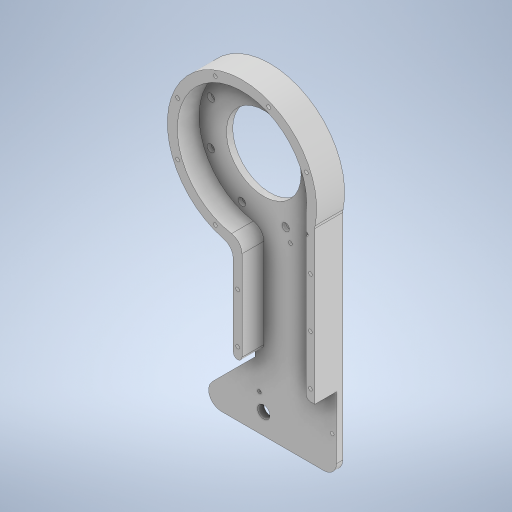
# Autodesk Inventor part: l_r_w2k_l__legparts_08(six)
Saved by Autodesk Inventor 2024.3 (Build 283343000, 343)
## iProperties
Created: 2024-10-20
Part Number: l_r_w2k_l__legparts_08(six)
Material: 一般
Document SubType Name: Modeling
Designer: 佐藤智貴
Density: 1 g/cm^3
Appearance: 既定
Mass: 466.511 g
Surface Area: 676.478 cm^2
Volume: 172.782 cm^3
Author: 佐藤智貴
Autodesk Inventor part; units mm, degrees
ref_plane "YZ Plane" through (0, 0, 0) normal (1, 0, 0) x (0, 1, 0)
ref_plane "XZ Plane" through (0, 0, 0) normal (0, 1, 0) x (-1, 0, 0)
ref_plane "XY Plane" through (0, 0, 0) normal (0, 0, 1) x (1, 0, 0)
sketch "スケッチ1" plane through (0, 0, 0) normal (0, 0, 1) x (1, 0, 0)
  circle A0 centre (0, 0) radius 60
  circle A1 centre (0, 0) radius 7
  dimension "d0" = 120
  dimension "d1" = 14
  constraints: 2 centre point, 1 coincident
  measures "d0" diameter of A0
  measures "d1" diameter of A1
extrude "押し出し1" add sketch "スケッチ1" along normal blind 5
sketch "スケッチ2" plane through (0, 0, 5) normal (0, 0, 1) x (1, 0, 0)
  circle A0 centre (0, 0) radius 46
  line L0 (0, 0) -> (0, 59.211)
  line L1 (0, 0) -> (-21.8609, 52.777)
  line L2 (0, 0) -> (27.8226, 47.8581)
  point P0 (-17.6034, 42.4985)
  point P1 (-42.4985, 17.6034)
  point P2 (-42.4985, -17.6034)
  point P3 (-17.6034, -42.4985)
  point P4 (17.6034, -42.4985)
  point P5 (42.4985, -17.6034)
  point P6 (42.4985, 17.6034)
  point P7 (17.6034, 42.4985)
  dimension "d4" = 92
  dimension "d5" = 22.5
  dimension "d8" = 360
  constraints: 6 end point, 1 coincident, 1 point on line, 1 vertical, 12 other
  measures "d5" angle of L1 L0
hole "穴1" at (-17.6034, 42.4985, 5) at (-42.4985, 17.6034, 5) at (-42.4985, -17.6034, 5) at (-17.6034, -42.4985, 5) at (17.6034, -42.4985, 5) at (42.4985, -17.6034, 5) at (42.4985, 17.6034, 5) at (17.6034, 42.4985, 5) direction (0, 0, -1) diameter 2.459 end through all
sketch "スケッチ4" plane through (0, 0, 0) normal (0, 0, -1) x (-1, 0, 0)
  line L0 (0, 0) -> (0, -80.557)
  circle A0 centre (0, 0) radius 60 projected
  line L1 (-58.5, 13.3323) -> (-58.5, -196.6677)
  line L2 (58.5, 13.3323) -> (58.5, -196.6677)
  line L3 (-58.5, -196.6677) -> (58.5, -196.6677)
  line L4 (-58.5, 13.3323) -> (-40.1274, -196.6677)
  line L5 (58.5, 13.3323) -> (40.1274, -196.6677)
  line L6 (11.2278, -149.3955) -> (58.5, -196.6677)
  line L7 (18.206, -156.3737) -> (-9.1224, -129.0453)
  line L8 (0, -80.557) -> (0, -138.1677)
  line L9 (7, -239.3448) -> (7, -80.557)
  line L10 (7, -80.557) -> (7, 0)
  line L11 (7, -239.3448) -> (7, -145.1677)
  circle A1 centre (0, 0) radius 7 projected
  point P0 (58.5, 13.3323)
  point P1 (55.2961, -23.2882)
  point P2 (-55.2961, -23.2882)
  point P3 (-58.5, -13.3323)
  point P4 (58.5, -13.3323)
  point P5 (58.5, 13.3323)
  point P6 (7, -136.3384)
  point P7 (7, -59.5903)
  point P8 (41.6055, -179.7732)
  point P9 (7, -196.6677)
  point P10 (7, -136.3384)
  point P11 (7, -145.1677)
  dimension "d21" = 58.5
  dimension "d23" = 117
  dimension "d24" = 210
  dimension "d25" = 210
  dimension "d56" = 0
  dimension "d89" = 85
  dimension "d90" = 85
  dimension "d207" = 45
  dimension "d208" = 7
  constraints: 24 end point, 6 point on line, 2 vertical, 1 horizontal alignment, 1 perpendicular, 3 other
  measures "d21" distance from line of L1 L0.start
  measures "d23" distance between parallel lines of L2 L1
  measures "d24" distance of L2.start L2.end
  measures "d25" distance of L1.start L1.end
  measures "d56" angle of L2 L0
  measures "d89" angle of L3 L5
  measures "d90" angle of L3 L4
  measures "d207" angle of L3 L6
  measures "d208" distance between parallel lines of L8 L9
extrude "押し出し3" add sketch "スケッチ4" against normal blind 5 contours A0 L10 L9 L7 L8 L0 | L0 L8 L7 L9 L3 L4 A0 | L4 L3 L1 A0 | L7 L6 L5 L3 L9 | L6 L3 L5
sketch "スケッチ15" plane through (0, 0, 5) normal (0, 0, 1) x (1, 0, 0)
  circle A0 centre (0, 0) radius 43.5
  circle A1 centre (0, 0) radius 12.5
  line L0 (0, 0) -> (-4.8577, 8.4138)
  line L1 (0, 0) -> (0, 11.0896)
  point P0 (-6.25, 10.8253)
  point P1 (6.25, 10.8253)
  point P2 (12.5, 0)
  point P3 (6.25, -10.8253)
  point P4 (-6.25, -10.8253)
  point P5 (-12.5, 0)
  dimension "d134" = 25
  dimension "d133" = 87
  dimension "d135" = 30
  dimension "d136" = 360
  constraints: 4 end point, 3 coincident, 1 centre point, 1 point on line, 1 vertical, 10 other
  measures "d133" diameter of A0
  measures "d135" angle of L1 L0
hole "穴6" at (-6.25, 10.8253, 5) at (-12.5, 0, 5) at (-6.25, -10.8253, 5) at (6.25, -10.8253, 5) at (12.5, 0, 5) at (6.25, 10.8253, 5) direction (0, 0, -1) diameter 2.459 end through all
sketch "スケッチ16" plane through (0, 0, 5) normal (0, 0, 1) x (1, 0, 0)
  circle A0 centre (0, 0) radius 10.2
  point P0 (0, 10.2)
  point P1 (-8.8335, -5.1)
  point P2 (8.8335, -5.1)
  dimension "d146" = 20.4
  dimension "d150" = 360
  constraints: 3 coincident, 1 vertical alignment, 6 other
hole "穴7" at (0, 10.2, 5) at (-8.8335, -5.1, 5) at (8.8335, -5.1, 5) direction (0, 0, -1) diameter 4 end through all
sketch "スケッチ17" plane through (0, 0, 5) normal (0, 0, 1) x (1, 0, 0)
  circle A0 centre (0, 0) radius 30
  dimension "d159" = 60
  constraints: 1 centre point, 1 coincident
  measures "d159" diameter of A0
extrude "押し出し10" cut sketch "スケッチ17" against normal blind 10
sketch "スケッチ18" plane through (0, 0, 5) normal (0, 0, 1) x (1, 0, 0)
  circle A0 centre (0, 0) radius 60
  circle A1 centre (0, 0) radius 52
  line L0 (-58.5, -196.6677) -> (-58.5, -13.3323) projected
  line L1 (-58.5, -196.6677) -> (-58.5, -13.3323)
  line L2 (58.5, -13.3323) -> (58.5, -196.6677) projected
  line L3 (-58.5, -13.3323) -> (58.5, -13.3323)
  line L4 (58.5, -13.3323) -> (58.5, -196.6677)
  line L5 (58.5, -196.6677) -> (-58.5, -196.6677)
  line L6 (-51.5, -287.8448) -> (-51.5, -12.1552)
  line L7 (51.5, -12.1552) -> (51.5, -287.8448)
  line L8 (-58.5, -13.3323) -> (-58.5, -196.6677) projected
  line L9 (-58.5, -136.6677) -> (-51.5, -136.6677)
  line L10 (51.5, -136.6677) -> (58.5, -136.6677)
  circle A2 centre (-42.4985, -17.6034) radius 1.2295 projected
  circle A3 centre (-42.4985, -17.6034) radius 4
  circle A4 centre (42.4985, -17.6034) radius 1.2295 projected
  circle A5 centre (42.4985, -17.6034) radius 4
  line L11 (0, 0) -> (0, -225.3683)
  line L12 (-7, 0) -> (-7, -225.3683)
  line L13 (-58.5, -136.6677) -> (58.5, -136.6677)
  line L14 (51.5, -12.1552) -> (51.5, -7.1937)
  point P0 (-51.5, -30.7855)
  point P1 (51.5, -30.7855)
  point P2 (51.5, -196.6677)
  point P3 (-51.5, -196.6677)
  point P4 (-51.5, -13.3323)
  point P5 (-50.2618, -13.3323)
  point P6 (50.2618, -13.3323)
  point P7 (51.5, -13.3323)
  point P8 (-58.5, -136.6677)
  point P9 (55, -136.6677)
  point P10 (58.5, -136.6677)
  point P11 (46.5, -15.5649)
  point P12 (46.5, -23.4688)
  point P13 (-41.5, -13.7301)
  point P14 (-41.5, -21.4768)
  point P15 (-44.7686, -14.31)
  point P16 (41.7749, -21.5374)
  point P17 (-7, -59.5903)
  point P18 (-7, -136.6677)
  point P19 (0, -136.6677)
  point P20 (0, -52)
  point P21 (46.5, -18.4539)
  point P22 (46.5, -20.5798)
  point P23 (-50.8134, -21.0476)
  point P24 (0, -60)
  point P25 (-7, -51.5267)
  point P26 (0, -196.6677)
  point P27 (-48.8824, -25.2093)
  point P28 (43.6939, -17.316)
  point P29 (43.1405, -18.652)
  point P30 (58.5, -136.6677)
  dimension "d162" = 120
  dimension "d163" = 8
  dimension "d164" = 7
  dimension "d165" = 7
  dimension "d168" = 60
  dimension "d169" = 60
  dimension "d193" = 8
  dimension "d194" = 8
  dimension "d224" = 7
  constraints: 24 end point, 4 perpendicular, 4 point on line, 3 centre point, 3 coincident, 3 collinear, 3 parallel, 2 vertical, 1 midpoint, 3 other
  measures "d162" diameter of A0
  measures "d164" distance between parallel lines of L0 L6
  measures "d165" distance between parallel lines of L2 L7
  measures "d168" distance between parallel lines of L5 L9
  measures "d169" distance from line of L5 point (55, -136.668)
  measures "d193" diameter of A3
  measures "d194" diameter of A5
  measures "d224" distance between parallel lines of L11 L12
extrude "押し出し11" add sketch "スケッチ18" along normal blind 17.5 contours A0 L3 L7 L14 A1 | L3 L6 A0 | L2 L10 L7 A0 | A0 L7 L3 | L6 L3 A1 L12 A0 | L12 A1 L11 A0 | A0 L11 L13 L12
sketch "スケッチ19" plane through (0, 0, 0) normal (0, 0, -1) x (-1, 0, 0)
  circle A0 centre (-17.6034, 42.4985) radius 1.2295 projected
  circle A1 centre (0, 0) radius 46
  circle A2 centre (-17.6034, 42.4985) radius 1.5
  circle A3 centre (-42.4985, 17.6034) radius 1.5
  circle A4 centre (-42.4985, -17.6034) radius 1.5
  circle A5 centre (-17.6034, -42.4985) radius 1.5
  circle A6 centre (17.6034, -42.4985) radius 1.5
  circle A7 centre (42.4985, -17.6034) radius 1.5
  circle A8 centre (42.4985, 17.6034) radius 1.5
  circle A9 centre (17.6034, 42.4985) radius 1.5
  circle A10 centre (-42.4985, -17.6034) radius 2.5
  circle A11 centre (42.4985, -17.6034) radius 2.5
  circle A12 centre (-55, -47.6034) radius 1.5
  line L0 (-58.5, -13.3323) -> (-58.5, -196.6677) projected
  line L1 (0, 0) -> (103.4806, 0)
  line L2 (103.4806, 0) -> (0, 0)
  line L3 (0, 0) -> (0, -101.4206)
  circle A13 centre (3.5, -47.6034) radius 1.5
  circle A14 centre (-55, -87.6034) radius 1.5
  circle A15 centre (3.5, -87.6034) radius 1.5
  circle A16 centre (-55, -127.6034) radius 1.5
  circle A17 centre (3.5, -127.6034) radius 1.5
  circle A18 centre (-55, -167.6034) radius 1.5
  circle A19 centre (3.5, -167.6034) radius 1.5
  point P0 (48.5, -239.3448)
  dimension "d172" = 3
  dimension "d175" = 360
  dimension "d177" = 5
  dimension "d178" = 5
  dimension "d179" = 3
  dimension "d180" = 3.5
  dimension "d181" = 30
  dimension "d185" = 58.5
  dimension "d188" = 40
  constraints: 18 centre point, 6 end point, 4 coincident, 2 horizontal, 2 vertical, 1 collinear, 34 other
  measures "d172" diameter of A2
  measures "d177" diameter of A11
  measures "d178" diameter of A10
  measures "d179" diameter of A12
  measures "d180" distance from line of L0 A12.centre
  measures "d181" vertical distance of A10.centre A12.centre
  measures "d185" distance of A12.centre A13.centre
  measures "d188" distance of A12.centre A14.centre
extrude "押し出し12" cut sketch "スケッチ19" against normal through all contours A0 A1 | A0 A1 A2 | A1 A0 | A0 A1 A2 | A9 A1 | A1 A9 | A3 A1 | A1 A3 | A8 A1 | A1 A8 | A4 A1 | A1 A4 | A5 A1 | A1 A5 | A7 A1 | A1 A7 | A6 A1 | A1 A6 | A12 | A14 | A15 | A16 | A17 | A18 | A19
sketch "スケッチ20" plane through (0, 0, 5) normal (0, 0, 1) x (1, 0, 0)
  line L0 (-58.5, -196.6677) -> (58.5, -196.6677) projected
  circle A0 centre (0, 0) radius 30 projected
  line L1 (58.5, -196.6677) -> (58.5, -136.6677) projected
  point P0 (0, -180)
  point P1 (0, -196.6677)
  point P2 (41.5, -184.0626)
  point P3 (48.5, -124.0626)
  point P4 (58.5, -13.3323)
  dimension "d205" = 180
  dimension "d223" = 58.5
  dimension "d246" = 58.5
  constraints: 3 other
  measures "d205" distance of point (0, -180) A0.centre
hole "穴8" at (0, -180, 5) direction (0, 0, -1) diameter 10 end through all
fillet "フィレット4" radius 10 2 edges at (-58.5, -196.6677, 2.5) (58.5, -196.6677, 2.5)
fillet "フィレット5" radius 10 3 edges at (-7, -59.5903, 11.25) (0, -52, 13.75) (58.5, -13.3323, 11.25)
fillet "フィレット6" radius 3.5 3 edges at (-7, -136.6677, 13.75) (0, -136.6677, 13.75) (51.5, -136.6677, 13.75)
sketch "スケッチ21" plane through (0, 0, 5) normal (0, 0, 1) x (1, 0, 0)
  circle A0 centre (-17.6034, 42.4985) radius 1.5 projected
  circle A1 centre (-17.6034, 42.4985) radius 3
  circle A2 centre (0, 0) radius 46
  circle A3 centre (-42.4985, 17.6034) radius 3
  circle A4 centre (-42.4985, -17.6034) radius 3
  circle A5 centre (-17.6034, -42.4985) radius 3
  circle A6 centre (17.6034, -42.4985) radius 3
  circle A7 centre (42.4985, -17.6034) radius 3
  circle A8 centre (42.4985, 17.6034) radius 3
  circle A9 centre (17.6034, 42.4985) radius 3
  dimension "d225" = 6
  dimension "d228" = 360
  constraints: 8 centre point, 2 coincident, 20 other
  measures "d225" diameter of A1
extrude "押し出し13" cut sketch "スケッチ21" against normal blind 3 contours A0 A2 | A0 A2 A1 | A2 A0 | A0 A2 A1 | A9 A2 | A2 A9 | A3 A2 | A2 A3 | A8 A2 | A2 A8 | A4 A2 | A2 A4 | A5 A2 | A2 A5 | A7 A2 | A2 A7 | A6 A2 | A2 A6
sketch "スケッチ22" plane through (0, 0, 22.5) normal (0, 0, 1) x (1, 0, 0)
  circle A0 centre (0, 0) radius 56
  circle A1 centre (0, 0) radius 60
  circle A2 centre (0, 0) radius 52
  circle A3 centre (-17.6034, 42.4985) radius 3 projected
  line L0 (0, 0) -> (-17.6034, 42.4985)
  line L1 (-17.6034, 42.4985) -> (-30.2265, 72.9733)
  point P0 (-21.4303, 51.7373)
  point P1 (-51.7373, 21.4303)
  point P2 (-51.7373, -21.4303)
  point P3 (-21.4303, -51.7373)
  point P4 (21.4303, -51.7373)
  point P5 (51.7373, -21.4303)
  point P6 (51.7373, 21.4303)
  point P7 (21.4303, 51.7373)
  dimension "d233" = 112
  dimension "d232" = 120
  dimension "d234" = 104
  dimension "d237" = 360
  constraints: 4 end point, 2 centre point, 2 coincident, 2 point on line, 12 other
  measures "d232" diameter of A1
  measures "d234" diameter of A2
hole "穴9" at (-21.4303, 51.7373, 22.5) at (-51.7373, 21.4303, 22.5) at (-51.7373, -21.4303, 22.5) at (-21.4303, -51.7373, 22.5) at (21.4303, -51.7373, 22.5) at (51.7373, -21.4303, 22.5) at (51.7373, 21.4303, 22.5) at (21.4303, 51.7373, 22.5) direction (0, 0, -1) diameter 3 end through all
equation "\"d25\" = d24"
equation "\"d90\" = d89"
equation "\"d194\" = d193"
